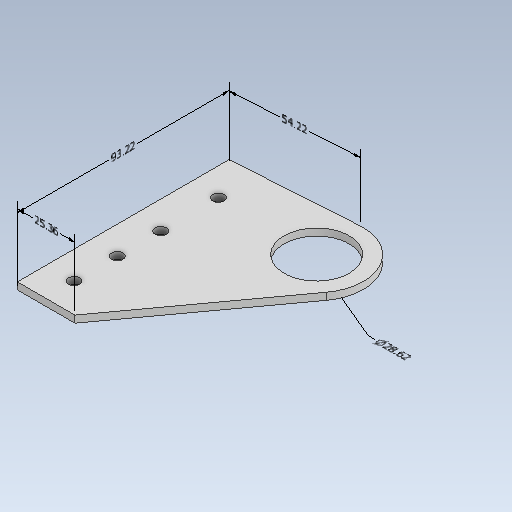
# Autodesk Inventor part: Bracket
Saved by Autodesk Inventor 2023 (Build 270158000, 158)
## iProperties
Created: 2023-02-11
Part Number: Bracket
Material: Generic
Document SubType Name: Modeling
Designer: coled
Density: 1 g/cm^3
Appearance: Default
Author: coled
Autodesk Inventor part; units mm, degrees
ref_plane "YZ Plane" through (0, 0, 0) normal (1, 0, 0) x (0, 1, 0)
ref_plane "XZ Plane" through (0, 0, 0) normal (0, 1, 0) x (-1, 0, 0)
ref_plane "XY Plane" through (0, 0, 0) normal (0, 0, 1) x (1, 0, 0)
sketch "Sketch1" plane through (0, 0, 0) normal (0, 1, 0) x (-1, 0, 0)
  line L0 (0, 0) -> (25.36, 0)
  line L1 (25.36, 0) -> (25.36, -93.22)
  line L2 (25.36, 0) -> (13.16, 0)
  line L3 (13.16, 0) -> (13.16, -10.27)
  line L4 (13.16, -10.27) -> (13.16, -12.77)
  circle A0 centre (13.16, -12.77) radius 2.5
  line L5 (13.16, -12.77) -> (13.16, -15.27)
  line L6 (13.16, -15.27) -> (13.16, -29.33)
  line L7 (13.16, -29.33) -> (13.16, -31.83)
  circle A1 centre (13.16, -31.83) radius 2.5
  line L8 (13.16, -31.83) -> (13.16, -34.33)
  line L9 (13.16, -34.33) -> (13.16, -48.39)
  line L10 (13.16, -48.39) -> (13.16, -50.89)
  circle A2 centre (13.16, -50.89) radius 2.5
  line L11 (13.16, -50.89) -> (13.16, -53.39)
  line L12 (13.16, -53.39) -> (13.16, -73.79)
  line L13 (13.16, -73.79) -> (13.16, -76.29)
  circle A3 centre (13.16, -76.29) radius 2.5
  line L14 (13.16, -76.29) -> (10.66, -76.29)
  line L15 (10.66, -76.29) -> (-15.82, -76.29)
  line L16 (-15.82, -76.29) -> (-30.095, -76.29)
  circle A4 centre (-30.095, -76.29) radius 14.31
  line L17 (-30.095, -76.29) -> (-30.095, -90.6)
  line L18 (-30.095, -90.6) -> (-30.095, -96.84)
  arc A5 (-46.7119, -64.1995) -> (-28.7399, -96.7953) centre (-30.095, -76.29) ccw
  line L19 (25.36, -93.22) -> (-28.7399, -96.7953)
  line L20 (0, 0) -> (-46.7119, -64.1995)
  dimension "d25" = 28.62
  dimension "d1" = 25.36
  dimension "d2" = 93.22
  dimension "d3" = 12.2
  dimension "d4" = 10.27
  dimension "d5" = 2.5
  dimension "d10" = 14.06
  dimension "d11" = 2.5
  dimension "d12" = 14.06
  dimension "d13" = 2.5
  dimension "d14" = 20.4
  dimension "d15" = 2.5
  dimension "d16" = 26.48
  dimension "d17" = 14.275
  dimension "d26" = 6.24
  constraints: 42 end point, 11 point on circle, 10 point on line, 6 coincident, 5 centre point, 5 vertical, 2 horizontal, 2 perpendicular, 2 tangent, 1 vertical alignment, 2 other
  measures "d1" distance of L0.start L0.end
  measures "d2" distance of L0.end L1.end
  measures "d3" distance of L0.end L2.end
  measures "d4" distance of L2.end L3.end
  measures "d5" distance of L3.end L4.end
  measures "d10" distance of L5.end L6.end
  measures "d11" distance of L6.end L7.end
  measures "d12" distance of L8.end L9.end
  measures "d13" distance of L9.end L10.end
  measures "d14" distance of L11.end L12.end
  measures "d15" distance of L12.end L13.end
  measures "d16" distance of L14.end L15.end
  measures "d17" distance of L15.end L16.end
  measures "d26" distance of L17.end L18.end
extrude "Extrusion2" add sketch "Sketch1" along normal blind 3.07 contours L0 L3 A0 L6 A1 L9 A2 L12 A3 L15 A4 L18 A5 L20 | L0 L1 L19 A5 L18 A4 L15 A3 L12 A2 L9 A1 L6 A0 L3
body "Solid2"
